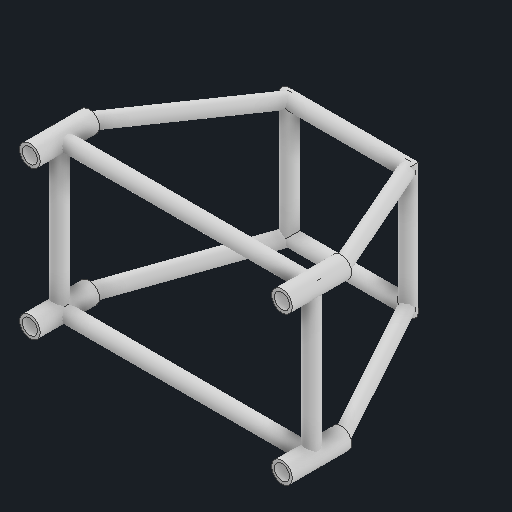
# Autodesk Inventor part: RCPlaneSkeletonFront2
Saved by Autodesk Inventor 2026.1 (Build 301233000, 233)
## iProperties
Created: 2026-03-16
Part Number: RCPlaneSkeletonFront2
Material: Generic
Document SubType Name: Modeling
Designer: morri
Density: 1 g/cm^3
Appearance: Default
Mass: 21.7529 g
Surface Area: 219.341 cm^2
Volume: 21.7529 cm^3
Author: morri
Autodesk Inventor part; units mm, degrees
ref_plane "YZ Plane" through (0, 0, 0) normal (1, 0, 0) x (0, 1, 0)
ref_plane "XZ Plane" through (0, 0, 0) normal (0, 1, 0) x (-1, 0, 0)
ref_plane "XY Plane" through (0, 0, 0) normal (0, 0, 1) x (1, 0, 0)
ref_plane "Work Plane1" through (22.5, 5, -45) normal (0, 1, 0) x (-1, 0, 0)
ref_plane "Work Plane2" through (0, 0, 10) normal (0, 1, 0) x (-1, 0, 0)
sketch "Sketch1" plane through (0, 0, 0) normal (0, 0, 1) x (1, 0, 0)
  circle A0 centre (0, 0) radius 3.5
  line L0 (0, 0) -> (85, 0) construction
  line L1 (85, 0) -> (85, 50) construction
  line L2 (85, 50) -> (0, 50) construction
  line L3 (0, 50) -> (0, 0) construction
  circle A1 centre (0, 50) radius 3.5
  circle A2 centre (85, 50) radius 3.5
  circle A3 centre (85, 0) radius 3.5
  dimension "d15" = 7
  dimension "d16" = 85
  dimension "d17" = 50
  dimension "d18" = 7
  dimension "d19" = 7
  dimension "d20" = 7
  constraints: 8 end point, 4 centre point, 4 coincident, 2 parallel, 1 horizontal, 1 perpendicular
  measures "d15" diameter of A0
  measures "d16" distance of L2.end L1.end
  measures "d17" distance of L1.end L0.end
  measures "d18" diameter of A1
  measures "d19" diameter of A2
  measures "d20" diameter of A3
extrude "Extrusion1" add sketch "Sketch1" along normal blind 20
sketch "Sketch2" plane through (0, 0, 0) normal (0, 0, 1) x (1, 0, 0)
  circle A0 centre (0, 0) radius 3.5 projected
  circle A1 centre (0, 0) radius 2.5
  circle A2 centre (0, 50) radius 3.5 projected
  circle A3 centre (0, 50) radius 2.5
  circle A4 centre (85, 50) radius 3.5 projected
  circle A5 centre (85, 50) radius 2.5
  circle A6 centre (85, 0) radius 3.5 projected
  circle A7 centre (85, 0) radius 2.5
  dimension "d23" = 5
  dimension "d24" = 5
  dimension "d25" = 5
  dimension "d26" = 5
  constraints: 4 centre point, 4 coincident
  measures "d23" diameter of A1
  measures "d24" diameter of A3
  measures "d25" diameter of A5
  measures "d26" diameter of A7
sketch3d "3D Sketch1"
  line L0 (0, 0, 0) -> (22.5, 5, -45)
  dimension "d0" = 50
  dimension "d1" = 85
  dimension "d2" = 50
  dimension "d3" = 45
  dimension "d4" = 5
  dimension "d5" = 22.5
  dimension "d6" = 40
  dimension "d7" = 40
  dimension "d8" = 40
  dimension "d38" = 10
  dimension "d39" = 50
  dimension "d40" = 85
  dimension "d41" = 50
sweep "Sweep1" add profiles "Sketch2" path "3D Sketch1" separate body contours A1
sketch3d "3D Sketch1 for Sweep2"
  line L0 (0, 50, 0) -> (22.5, 45, -45)
  dimension "d0" = 50
  dimension "d1" = 85
  dimension "d2" = 50
  dimension "d3" = 45
  dimension "d4" = 5
  dimension "d5" = 22.5
  dimension "d6" = 40
  dimension "d7" = 40
  dimension "d8" = 40
  dimension "d38" = 10
  dimension "d39" = 50
  dimension "d40" = 85
  dimension "d41" = 50
sweep "Sweep2" add profiles "Sketch2" path "3D Sketch1 for Sweep2" separate body contours A3
sketch3d "3D Sketch1 for Sweep3"
  line L0 (85, 50, 0) -> (62.5, 45, -45)
  dimension "d0" = 50
  dimension "d1" = 85
  dimension "d2" = 50
  dimension "d3" = 45
  dimension "d4" = 5
  dimension "d5" = 22.5
  dimension "d6" = 40
  dimension "d7" = 40
  dimension "d8" = 40
  dimension "d38" = 10
  dimension "d39" = 50
  dimension "d40" = 85
  dimension "d41" = 50
sweep "Sweep3" add profiles "Sketch2" path "3D Sketch1 for Sweep3" separate body contours A5
sketch3d "3D Sketch1 for Sweep4"
  line L0 (85, 0, 0) -> (62.5, 5, -45)
  dimension "d0" = 50
  dimension "d1" = 85
  dimension "d2" = 50
  dimension "d3" = 45
  dimension "d4" = 5
  dimension "d5" = 22.5
  dimension "d6" = 40
  dimension "d7" = 40
  dimension "d8" = 40
  dimension "d38" = 10
  dimension "d39" = 50
  dimension "d40" = 85
  dimension "d41" = 50
sweep "Sweep4" add profiles "Sketch2" path "3D Sketch1 for Sweep4" separate body contours A7
sketch "Sketch3" plane through (22.5, 5, -45) normal (0, 1, 0) x (-1, 0, 0)
  line L0 (-2.5, 0) -> (2.5, 0) projected
  circle A0 centre (0, 0) radius 2.5
  point P0 (22.5, 45)
  dimension "d35" = 5
  constraints: 1 centre point, 1 midpoint
  measures "d35" diameter of A0
sketch3d "3D Sketch1 for Sweep5"
  line L0 (22.5, 5, -45) -> (22.5, 45, -45)
  line L1 (22.5, 45, -45) -> (62.5, 45, -45)
  line L2 (62.5, 45, -45) -> (62.5, 5, -45)
  line L3 (62.5, 5, -45) -> (22.5, 5, -45)
  dimension "d0" = 50
  dimension "d1" = 85
  dimension "d2" = 50
  dimension "d3" = 45
  dimension "d4" = 5
  dimension "d5" = 22.5
  dimension "d6" = 40
  dimension "d7" = 40
  dimension "d8" = 40
  dimension "d38" = 10
  dimension "d39" = 50
  dimension "d40" = 85
  dimension "d41" = 50
sweep "Sweep5" add profiles "Sketch3" path "3D Sketch1 for Sweep5" separate body
sketch "Sketch4" plane through (0, 0, 10) normal (0, 1, 0) x (-1, 0, 0)
  circle A0 centre (0, 0) radius 2.5
  point P0 (0, -10)
  dimension "d42" = 5
  constraints: 1 centre point
  measures "d42" diameter of A0
sketch3d "3D Sketch1 for Sweep6"
  line L0 (0, 0, 10) -> (0, 50, 10)
  line L1 (0, 50, 10) -> (85, 50, 10)
  line L2 (85, 50, 10) -> (85, 0, 10)
  line L3 (85, 0, 10) -> (0, 0, 10)
  dimension "d0" = 50
  dimension "d1" = 85
  dimension "d2" = 50
  dimension "d3" = 45
  dimension "d4" = 5
  dimension "d5" = 22.5
  dimension "d6" = 40
  dimension "d7" = 40
  dimension "d8" = 40
  dimension "d38" = 10
  dimension "d39" = 50
  dimension "d40" = 85
  dimension "d41" = 50
sweep "Sweep6" add profiles "Sketch4" path "3D Sketch1 for Sweep6" separate body
sketch "Sketch5" plane through (0, 0, 20) normal (0, 0, 1) x (1, 0, 0)
  line L0 (2.5, 47.5) -> (-2.5, 52.5) projected
  line L1 (82.5, 47.5) -> (87.5, 52.5) projected
  line L2 (82.5, 2.5) -> (87.5, -2.5) projected
  point P0 (0, 0)
  point P1 (0, 0)
  point P2 (0, 50)
  point P3 (85, 50)
  point P4 (85, 0)
  constraints: 3 midpoint, 1 coincident
hole "Hole2" at (0, 50, 20) at (85, 50, 20) at (85, 0, 20) at (0, 0, 20) direction (0, 0, -1) diameter 5.1 depth 15 bodies 1 7
equation "\"fitTol\" = 0.1"
body "Solid1"
body "Solid2"
body "Solid4"
body "Solid5"
body "Solid6"
body "Solid7"
body "Solid8"
body "Solid9"
